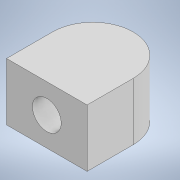
# Autodesk Inventor part: SUPPORT_POULIE
Saved by Autodesk Inventor 2020 (Build 240168000, 168)
## iProperties
Created: 2020-06-12
Part Number: SUPPORT_POULIE
Material: Generic
Document SubType Name: Modeling
Designer: Admin
Density: 1 g/cm^3
Appearance: Default
Author: Admin
Autodesk Inventor part; units mm, degrees
ref_plane "YZ Plane" through (0, 0, 0) normal (1, 0, 0) x (0, 1, 0)
ref_plane "XZ Plane" through (0, 0, 0) normal (0, 1, 0) x (-1, 0, 0)
ref_plane "XY Plane" through (0, 0, 0) normal (0, 0, 1) x (1, 0, 0)
sketch "Sketch1" plane through (0, 0, 0) normal (0, 1, 0) x (-1, 0, 0)
  line L0 (0, -8) -> (0, 0)
  line L1 (0, 0) -> (14, 0)
  line L2 (14, 0) -> (14, -8)
  arc A0 (0, -8) -> (14, -8) centre (7, -8) ccw
  dimension "d0" = 14
  dimension "d1" = 7
  dimension "d2" = 8
  constraints: 6 end point, 2 perpendicular, 2 point on circle, 1 centre point, 1 vertical
  measures "d0" distance of L0.end L1.end
  measures "d1" radius of A0
  measures "d2" distance from line of L1 A0.centre
extrude "Extrusion1" add sketch "Sketch1" along normal blind 10
sketch "Sketch2" plane through (-14, 0, 0) normal (0, 0, 1) x (1, 0, 0)
  circle A0 centre (7, 5) radius 2.5
  line L0 (0, 0) -> (14, 0) projected
  line L1 (0, 0) -> (0, 10) projected
  dimension "d5" = 5
  dimension "d6" = 5
  dimension "d7" = 7
  constraints: 1 centre point
  measures "d5" diameter of A0
  measures "d6" distance from line of A0.centre L0
  measures "d7" distance from line of A0.centre L1
extrude "Extrusion2" cut sketch "Sketch2" against normal through all
chamfer "Chamfer1" distance 2 angle 45 1 edges at (-9.5, 5.0035, -14.5383)
body "Solid1"
